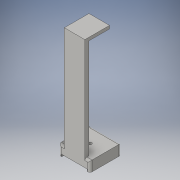
# Autodesk Inventor part: IDISCO-Sampleholder-12mm-60mm
Saved by Autodesk Inventor 2016 (Build 200138000, 138)
## iProperties
Created: 2018-07-25
Part Number: IDISCO-Sampleholder-12mm-60mm
Material: Generic
Document SubType Name: Modeling
Designer: voigt
Density: 1 g/cm^3
Appearance: Default
Author: voigt
Autodesk Inventor part; units mm, degrees
ref_plane "YZ Plane" through (0, 0, 0) normal (1, 0, 0) x (0, 1, 0)
ref_plane "XZ Plane" through (0, 0, 0) normal (0, 1, 0) x (-1, 0, 0)
ref_plane "XY Plane" through (0, 0, 0) normal (0, 0, 1) x (1, 0, 0)
sketch "Sketch1" plane through (0, 0, 0) normal (0, 0, 1) x (1, 0, 0)
  line L0 (0, 21) -> (0, -21) construction
  line L1 (-21, 0) -> (21, 0) construction
  line L2 (-15, 15) -> (15, 15)
  line L3 (15, 15) -> (15, -15)
  line L4 (15, -15) -> (-15, -15)
  line L5 (-15, -15) -> (-15, 15)
  point P0 (0, 0)
  dimension "d0" = 30
  dimension "d1" = 30
  constraints: 8 end point, 2 parallel, 1 horizontal, 1 perpendicular, 2 other
  measures "d0" distance of L2.end L3.end
  measures "d1" distance of L2.start L2.end
extrude "Extrusion1" add sketch "Sketch1" along normal blind 10
sketch "Sketch3" plane through (0, 0, 10) normal (0, 0, 1) x (1, 0, 0)
  line L0 (15, 15) -> (-15, 15) construction
  line L1 (-15, 15) -> (-15, -15) construction
  line L2 (-15, -15) -> (15, -15) construction
  line L3 (15, -15) -> (15, 15) construction
  line L4 (0, 21) -> (0, -21) construction
  line L5 (-21, 0) -> (21, 0) construction
  line L6 (-15, -15) -> (15, -15) projected
  line L7 (-10, -11) -> (10, -11)
  line L8 (10, -11) -> (10, -15)
  line L9 (10, -15) -> (-10, -15)
  line L10 (-10, -15) -> (-10, -11)
  point P0 (0, 0)
  dimension "d29" = 20
  dimension "d30" = 4
  constraints: 8 end point, 2 parallel, 1 horizontal, 1 perpendicular, 1 point on line, 1 other
  measures "d29" distance between parallel lines of L8 L10
  measures "d30" distance between parallel lines of L2 L7
extrude "Extrusion2" add sketch "Sketch3" along normal blind 100
sketch "Sketch5" plane through (0, 0, 0) normal (0, 0, -1) x (-1, 0, 0)
  point P0 (0, 0)
  point P1 (0, 0)
  constraints: 1 coincident
hole "Hole1" at (0, 0, 0) direction (0, 0, 1) diameter 3.3 end through all
sketch "Sketch7" plane through (-15, 15, 0) normal (0, 1, 0) x (1, 0, 0)
  line L0 (30, -10) -> (0, -10) construction
  line L1 (30, 0) -> (30, -10) construction
  line L2 (0, 0) -> (30, 0) construction
  line L3 (0, 0) -> (0, -10) construction
  line L4 (30, 0) -> (0, 0) projected
  line L5 (2.5, 0) -> (27.5, 0)
  line L6 (27.5, 0) -> (27.5, -2)
  line L7 (27.5, -2) -> (2.5, -2)
  line L8 (2.5, -2) -> (2.5, 0)
  line L9 (15, 22) -> (15, -132) construction
  point P0 (15, 0)
  dimension "d23" = 2
  dimension "d24" = 25
  constraints: 8 end point, 2 parallel, 1 horizontal, 1 perpendicular, 1 point on line, 1 other
  measures "d23" distance of L5.end L6.end
  measures "d24" distance between parallel lines of L6 L8
extrude "Extrusion5" cut sketch "Sketch7" against normal up to next
fillet "Fillet1" radius 2 7 edges at (0, 15, 10) (12.5, -15, 10) (-12.5, -15, 10) (-15, -15, 5) (-15, 15, 5) (15, 15, 5) (15, -15, 5)
sketch "Sketch8" plane through (-10, -11, 10) normal (0, 1, 0) x (1, 0, 0)
  line L0 (0, 0) -> (20, 0) construction
  line L1 (0, 0) -> (0, -100) construction
  line L2 (20, -100) -> (0, -100) construction
  line L3 (20, 0) -> (20, -100) construction
  line L4 (0, -100) -> (20, -100)
  line L5 (20, -100) -> (20, -97)
  line L6 (20, -97) -> (0, -97)
  line L7 (0, -97) -> (0, -100)
  point P0 (10, 10)
  dimension "d31" = 3
  constraints: 8 end point, 2 parallel, 1 horizontal, 1 perpendicular, 1 point on line
  measures "d31" distance between parallel lines of L2 L6
extrude "Extrusion6" add sketch "Sketch8" along normal blind 20
sketch "Sketch9" plane through (-10, -11, 10) normal (0, 1, 0) x (1, 0, 0)
  point P0 (10, 10)
body "Solid1"
